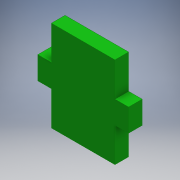
# Autodesk Inventor part: abajo1
Saved by Autodesk Inventor 2018 (Build 220112000, 112)
## iProperties
Created: 2020-03-13
Part Number: abajo1
Material: Genérico
Document SubType Name: Modeling
Designer: joser
Density: 1 g/cm^3
Appearance: Verde oscuro
Author: joser
Autodesk Inventor part; units mm, degrees
ref_plane "YZ Plane" through (0, 0, 0) normal (1, 0, 0) x (0, 1, 0)
ref_plane "XZ Plane" through (0, 0, 0) normal (0, 1, 0) x (-1, 0, 0)
ref_plane "XY Plane" through (0, 0, 0) normal (0, 0, 1) x (1, 0, 0)
sketch "Boceto1" plane through (0, 0, 0) normal (0, 1, 0) x (-1, 0, 0)
  line L0 (0, 0) -> (-14, 0)
  line L1 (-17, -7.5) -> (-17, -12.5)
  line L2 (-14, -20) -> (0, -20)
  line L3 (3, -12.5) -> (3, -7.5)
  line L4 (3, -12.5) -> (0, -12.5)
  line L5 (3, -7.5) -> (0, -7.5)
  line L6 (-14, -12.5) -> (-17, -12.5)
  line L7 (-14, -7.5) -> (-17, -7.5)
  line L8 (0, -20) -> (0, -12.5)
  line L9 (0, -7.5) -> (0, 0)
  line L10 (-14, -20) -> (-14, -12.5)
  line L11 (-14, -7.5) -> (-14, 0)
  dimension "d0" = 20
  dimension "d1" = 20
  dimension "d4" = 3
  dimension "d5" = 5
  constraints: 24 end point, 7 perpendicular, 5 equal length, 2 parallel, 2 point on line, 2 vertical, 1 coincident, 1 horizontal
  measures "d0" distance between parallel lines of L1 L3
  measures "d1" distance between parallel lines of L2 L0
  measures "d4" distance between parallel lines of L9 L3
  measures "d5" distance of L3.start L3.end
extrude "Extrusión1" add sketch "Boceto1" along normal blind 3
